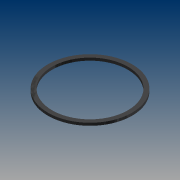
# Autodesk Inventor part: washer
Saved by Autodesk Inventor 2015 (Build 190159000, 159)
## iProperties
Created: 2021-03-23
Part Number: washer
Material: Rubber, Silicone
Document SubType Name: Modeling
Designer: Diptanshu Das
Density: 1.25 g/cm^3
Appearance: Rubber - Black - Version 1.1
Author: Diptanshu Das
Autodesk Inventor part; units mm, degrees
ref_plane "YZ Plane" through (0, 0, 0) normal (1, 0, 0) x (0, 1, 0)
ref_plane "XZ Plane" through (0, 0, 0) normal (0, 1, 0) x (-1, 0, 0)
ref_plane "XY Plane" through (0, 0, 0) normal (0, 0, 1) x (1, 0, 0)
sketch "Sketch1" plane through (0, 0, 0) normal (0, 0, 1) x (1, 0, 0)
  circle A0 centre (0, 0) radius 40
  circle A1 centre (0, 0) radius 36
  dimension "d0" = 80
  dimension "d1" = 72
  constraints: 2 centre point, 2 coincident
  measures "d0" diameter of A0
  measures "d1" diameter of A1
extrude "Extrusion1" add sketch "Sketch1" along normal blind 2.5
body "Solid1"
